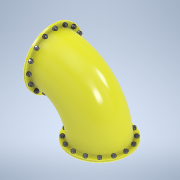
# Autodesk Inventor part: pipe_bend
Saved by Autodesk Inventor 2022 (Build 260153000, 153)
## iProperties
Created: 2021-12-16
Part Number: pipe_bend
Material: Steel
Document SubType Name: Modeling
Designer: jpc
Density: 7.85 g/cm^3
Appearance: Steel Galvanized
Mass: 2.14484e+06 g
Surface Area: 119776 cm^2
Volume: 273228 cm^3
Author: jpc
Autodesk Inventor part; units mm, degrees
ref_plane "YZ Plane" through (0, 0, 0) normal (1, 0, 0) x (0, 1, 0)
ref_plane "XZ Plane" through (0, 0, 0) normal (0, 1, 0) x (-1, 0, 0)
ref_plane "XY Plane" through (0, 0, 0) normal (0, 0, 1) x (1, 0, 0)
sketch "cross_section" plane through (0, 0, 0) normal (0, 1, 0) x (-1, 0, 0)
  circle A0 centre (0, 0) radius 500
  circle A1 centre (0, 0) radius 450
  dimension "dia_out" = 1000
  dimension "dia_in" = 900
  constraints: 2 centre point, 2 coincident
  measures "dia_out" diameter of A0
  measures "dia_in" diameter of A1
sketch "curved_midline" plane through (0, 0, 0) normal (0, 0, 1) x (1, 0, 0)
  arc A0 (1000, 1000) -> (0, 0) centre (1000, 0) ccw
  line L0 (0, 0) -> (1000, 0) construction
  line L1 (1000, 0) -> (1000, 1000) construction
  dimension "d4" = 1000
  constraints: 4 end point, 2 point on circle, 1 centre point, 1 horizontal, 1 perpendicular
  measures "d4" distance of L0.end L1.end
sketch "straight_midline" plane through (0, 0, 0) normal (0, 0, 1) x (1, 0, 0)
  line L0 (0, 0) -> (0, 10000)
  dimension "len" = 10000
  constraints: 2 end point, 1 vertical
  measures "len" distance of L0.start L0.end
sweep "Sweep" add profiles "cross_section" path "curved_midline"
sketch "Sketch4" plane through (0, 0, 0) normal (0, -1, 0) x (1, 0, 0)
  circle A0 centre (0, 0) radius 600
  circle A1 centre (0, 0) radius 450 projected
  dimension "endcap_dia" = 1200
  constraints: 1 centre point, 1 coincident
  measures "endcap_dia" diameter of A0
extrude "Endcap" add sketch "Sketch4" against normal blind 50
ref_plane "Midplane" through (1000, 0, 0) normal (-0.7071068, -0.7071068, 0) x (0, 0, -1)
chamfer "Chamfer" distance 12.5 angle 45 1 edges at (-600, 0, 0)
sketch "Sketch7" plane through (0, 50, 0) normal (0, 1, 0) x (1, 0, 0)
  circle A0 centre (0, 0) radius 600 construction
  circle A1 centre (0, 0) radius 600 construction
  line L0 (-600, 0) -> (-499.1664, 0) construction
  circle A2 centre (-549.5832, 0) radius 25.2084
  arc A3 (0.625, -449.9996) -> (0.625, 449.9996) centre (0, 0) ccw projected
  dimension "d27" = 100.8336
  dimension "d28" = 50.4168
  constraints: 2 end point, 2 vertical alignment, 1 centre point, 1 horizontal, 1 horizontal alignment, 1 midpoint, 2 other
  measures "d27" distance of L0.start L0.end
  measures "d28" diameter of A2
extrude "Hole" cut sketch "Sketch7" against normal through all
pattern_circular "Holes" count 16 over 360 about axis through (0, -10, 0) along (0, 1, 0) of "Hole"
mirror "MirroredFeatures" about plane through (1000, 0, 0) normal (-0.7071068, -0.7071068, 0) of "Hole", "Holes", "Endcap", "Chamfer"
sketch "Sketch8" plane through (0, 50, 0) normal (0, 1, 0) x (1, 0, 0)
  circle A0 centre (-549.5832, 0) radius 25.2084 construction
  circle A1 centre (-549.5832, 0) radius 37.8126 construction
  circle A2 centre (0, 0) radius 587.5 construction
  line L0 (-587.5, 0) -> (-568.5416, 32.8369)
  line L1 (-568.5416, 32.8369) -> (-530.6248, 32.8369)
  line L2 (-530.6248, 32.8369) -> (-511.6664, 0)
  line L3 (-511.6664, 0) -> (-530.6248, -32.8369)
  line L4 (-530.6248, -32.8369) -> (-568.5416, -32.8369)
  line L5 (-568.5416, -32.8369) -> (-587.5, 0)
  dimension "d34" = 50.4168
  dimension "d35" = 75.6252
  constraints: 12 end point, 2 coincident, 1 centre point, 1 horizontal, 1 horizontal alignment, 14 other
  measures "d34" diameter of A0
  measures "d35" diameter of A1
extrude "BoltHead" add sketch "Sketch8" along normal blind 37.5 separate body
sketch "Sketch9" plane through (0, 50, 0) normal (0, -1, 0) x (1, 0, 0)
  circle A0 centre (-549.5832, 0) radius 25.2084 projected
  point P0 (0, 0)
extrude "BoltThreadHalf" add sketch "Sketch9" along normal blind 45 bodies 2
pattern_circular "BoltHalves" count 16 over 360 about axis through (0, -10, 0) along (0, 1, 0) bodies 2
mirror "MirroredBolts" about plane through (1000, 0, 0) normal (-0.7071068, -0.7071068, 0) bodies 2
sketch "Sketch10" plane through (912.5, 1530.6248, 32.8369) normal (-1, 0, 0) x (0, 0, 1)
  circle A0 centre (-32.8369, 18.9584) radius 25.2084 projected
  point P0 (-32.8369, -1530.6248)
extrude "ExtraThread" add sketch "Sketch10" along normal blind 22.5 bodies 2
chamfer "ThreadChamfer" distance 6.25 angle 45 1 edges at (890, 1549.5832, -25.2084)
pattern_circular "BoltNuts" count 16 over 360 about axis through (950, 1000, 0) along (1, 0, 0) of "ExtraThread", "ThreadChamfer" bodies 2
mirror "Mirror4" about plane through (0, 0, 0) normal (1, 0, 0) remove original yes bodies 2 1
equation "\"d4\" = dia_out"
equation "\"endcap_dia\" = 1.2 * dia_out"
equation "\"endcap_thick\" = -0.5 * dia_in + 0.5 * dia_out"
equation "\"d28\" = 0.5 * d27"
equation "\"d35\" = 1.5 * d34"
equation "\"bolt_thick\" = 0.75 * endcap_thick"
equation "\"d38\" = 0.9 * endcap_thick"
equation "\"d43\" = 0.45 * endcap_thick"
equation "\"d48\" = 0.125 * endcap_thick"
equation "\"d24\" = 0.25 * endcap_thick"
